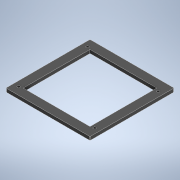
# Autodesk Inventor part: middleplate
Saved by Autodesk Inventor 2022 (Build 260153000, 153)
## iProperties
Created: 2022-01-15
Part Number: middleplate
Material: ABS Plastic
Document SubType Name: Modeling
Designer: Sergey
Density: 1.06 g/cm^3
Appearance: Generic
Author: Sergey
Autodesk Inventor part; units mm, degrees
ref_plane "YZ Plane" through (0, 0, 0) normal (1, 0, 0) x (0, 1, 0)
ref_plane "XZ Plane" through (0, 0, 0) normal (0, 1, 0) x (-1, 0, 0)
ref_plane "XY Plane" through (0, 0, 0) normal (0, 0, 1) x (1, 0, 0)
sketch "Sketch1" plane through (0, 0, 0) normal (0, 1, 0) x (-1, 0, 0)
  line L0 (1.2, 50) -> (1.2, 66.5)
  arc A0 (2.2, 73.8) -> (1.2, 72.8) centre (2.2, 72.8) ccw
  line L1 (1.2, 67.5) -> (1.2, 72.8)
  line L2 (1.2, 66.5) -> (1.2, 67.5)
  line L3 (7.5, 73.8) -> (8.5, 73.8)
  line L4 (2.2, 73.8) -> (7.5, 73.8)
  line L5 (8.5, 73.8) -> (25, 73.8)
  arc A1 (1.2, -22.8) -> (2.2, -23.8) centre (2.2, -22.8) ccw
  line L6 (1.2, -22.8) -> (1.2, -17.5)
  line L7 (7.5, -23.8) -> (2.2, -23.8)
  line L8 (8.5, -23.8) -> (7.5, -23.8)
  line L9 (25, -23.8) -> (8.5, -23.8)
  line L10 (1.2, -16.5) -> (1.2, 0)
  line L11 (1.2, -17.5) -> (1.2, -16.5)
  line L12 (97.8, -23.8) -> (92.5, -23.8)
  line L13 (92.5, -23.8) -> (91.5, -23.8)
  line L14 (91.5, -23.8) -> (75, -23.8)
  line L15 (98.8, -17.5) -> (98.8, -22.8)
  arc A2 (97.8, -23.8) -> (98.8, -22.8) centre (97.8, -22.8) ccw
  line L16 (98.8, -16.5) -> (98.8, -17.5)
  line L17 (98.8, 0) -> (98.8, -16.5)
  line L18 (91.5, 73.8) -> (92.5, 73.8)
  line L19 (75, 73.8) -> (91.5, 73.8)
  line L20 (92.5, 73.8) -> (97.8, 73.8)
  arc A3 (98.8, 72.8) -> (97.8, 73.8) centre (97.8, 72.8) ccw
  line L21 (98.8, 72.8) -> (98.8, 67.5)
  line L22 (98.8, 66.5) -> (98.8, 50)
  line L23 (98.8, 67.5) -> (98.8, 66.5)
  line L24 (1.2, 0) -> (1.2, 50)
  line L25 (25, -23.8) -> (75, -23.8)
  line L26 (98.8, 0) -> (98.8, 50)
  line L27 (75, 73.8) -> (25, 73.8)
  circle A4 centre (7.135, 62.465) radius 1.45
  circle A5 centre (7.135, -11.195) radius 1.45
  circle A6 centre (92.865, 65.005) radius 1.45
  circle A7 centre (92.865, -15.005) radius 1.45
  constraints: 56 end point, 8 centre point, 8 point on circle, 2 collinear, 1 perpendicular, 1 vertical
extrude "Extrusion1" add sketch "Sketch1" along normal blind 4
sketch "Sketch2" plane through (0, 4, 0) normal (0, 1, 0) x (1, 0, 0)
  line L0 (-98.8, 22.8) -> (-98.8, -72.8) projected
  arc A0 (-98.8, -72.8) -> (-97.8, -73.8) centre (-97.8, -72.8) ccw projected
  line L1 (-97.8, -73.8) -> (-2.2, -73.8) projected
  arc A1 (-2.2, -73.8) -> (-1.2, -72.8) centre (-2.2, -72.8) ccw projected
  line L2 (-1.2, -72.8) -> (-1.2, 22.8) projected
  arc A2 (-1.2, 22.8) -> (-2.2, 23.8) centre (-2.2, 22.8) ccw projected
  line L3 (-2.2, 23.8) -> (-97.8, 23.8) projected
  arc A3 (-97.8, 23.8) -> (-98.8, 22.8) centre (-97.8, 22.8) ccw projected
  circle A4 centre (-92.865, -65.005) radius 1.45 projected
  circle A5 centre (-92.865, 15.005) radius 1.45 projected
  circle A6 centre (-7.135, -62.465) radius 1.45 projected
  circle A7 centre (-7.135, 11.195) radius 1.45 projected
  line L4 (-97.8, -72.8) -> (-2.2, 22.8)
  line L5 (-11.2, -63.8) -> (-88.8, -63.8)
  line L6 (-88.8, -63.8) -> (-88.8, 13.8)
  line L7 (-88.8, 13.8) -> (-11.2, 13.8)
  line L8 (-11.2, 13.8) -> (-11.2, -63.8)
  line L9 (-11.2, -63.8) -> (-88.8, 13.8) construction
  line L10 (-88.8, -63.8) -> (-11.2, 13.8) construction
  point P0 (0, 0)
  point P1 (-50, -25)
  dimension "d4" = 10
  dimension "d5" = 10
  constraints: 14 end point, 3 midpoint, 2 parallel, 1 horizontal, 1 perpendicular
  measures "d4" distance between parallel lines of L0 L6
  measures "d5" distance between parallel lines of L1 L5
extrude "Extrusion2" cut sketch "Sketch2" against normal blind 4 contours L6 L7 L4 | L4 L8 L5
body "Solid1"
